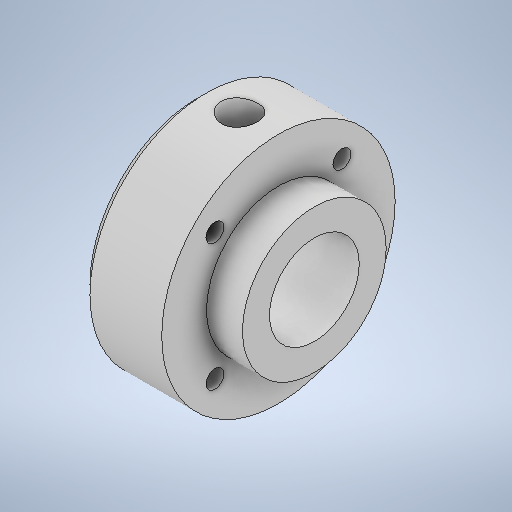
# Autodesk Inventor part: 08
Saved by Autodesk Inventor 2025.1 (Build 291241000, 241)
## iProperties
Created: 2024-09-17
Part Number: 08
Material: Generisch
Document SubType Name: Modeling
Designer: ffogue
Density: 1 g/cm^3
Appearance: Vorgabe
Author: ffogue
Autodesk Inventor part; units mm, degrees
ref_plane "YZ Plane" through (0, 0, 0) normal (1, 0, 0) x (0, 1, 0)
sketch "Sketch1" plane through (0, 0, 0) normal (0, 0, 1) x (1, 0, 0)
  line L0 (0, 0) -> (0, 13)
  line L1 (0, 13) -> (9, 13)
  line L2 (9, 13) -> (9, 8)
  line L3 (9, 8) -> (13, 8)
  line L4 (13, 8) -> (13, 0)
  line L5 (13, 0) -> (0, 0)
  dimension "d0" = 16
  dimension "d1" = 9
  dimension "d2" = 4
  dimension "d3" = 26
  constraints: 12 end point, 5 perpendicular, 1 vertical
  measures "d0" diameter of L3 L5
  measures "d1" distance of L0.end L1.end
  measures "d2" distance of L2.end L3.end
  measures "d3" diameter of L1 L5
revolve "Revolution1" add sketch "Sketch1" angle 360 about axis through (13, 0, 0) along (-1, 0, 0)
sketch "Sketch2" plane through (0, 0, 0) normal (-1, 0, 0) x (0, 0, 1)
  line L0 (0, 0) -> (7.0711, 7.0711) construction
  line L1 (0, 0) -> (13, 0) construction
  circle A0 centre (0, 0) radius 13 projected
  circle A1 centre (0, 0) radius 10 construction
  dimension "d6" = 20
  dimension "d5" = 45
  constraints: 4 end point, 2 horizontal alignment, 1 coincident, 1 horizontal, 4 other
  measures "d5" angle of L1 L0
hole "Hole1" at (0, 7.0711, 7.0711) direction (1, 0, 0) diameter 2 depth 9
pattern_circular "Circular Pattern1" count 4 over 360 about axis through (4.5, 0, 0) along (-1, 0, 0) of "Hole1"
sketch "Sketch3" plane through (0, 0, 0) normal (-1, 0, 0) x (0, 0, 1)
  circle A0 centre (0, 0) radius 13 projected
  point P0 (0, 0)
  constraints: 1 coincident
hole "Hole2" at (0, 0, 0) direction (1, 0, 0) diameter 10 depth 13
chamfer "Chamfer1" distance 1 angle 45 1 edges at (0, -13, 0)
ref_plane "Work Plane1" through (0, 0, 0) normal (0, 1, 0) x (-1, 0, 0)
sketch "Sketch4" plane through (0, 0, 0) normal (0, 1, 0) x (-1, 0, 0)
  line L0 (-13, -5) -> (-13, 5) projected
  line L1 (-13, -8) -> (-13, 8) projected
  line L2 (-7, 7) -> (-4.8162, 13)
  line L3 (-9, 13) -> (-1, 13) projected
  line L4 (-13, 5) -> (0, 5) projected
  point P0 (0, 0)
  dimension "d28" = 20
  dimension "d29" = 2
  dimension "d34" = 2
  constraints: 3 end point, 1 point on line
  measures "d28" angle of L1 L2
  measures "d29" horizontal distance of L3.start L2.start
  measures "d34" distance from line of L4 L2.start
ref_plane "Work Plane2" through (0, 0, 12.5) normal (0, 0, 1) x (1, 0, 0)
sketch "Sketch5" plane through (0, 0, 12.5) normal (0, 0, 1) x (1, 0, 0)
  circle A0 centre (4.8162, 0) radius 2
  point P0 (0, 0)
  dimension "d31" = 4
  constraints: 1 centre point, 1 coincident
  measures "d31" diameter of A0
sweep "Sweep1" cut profiles "Sketch5" path "Sketch4" path curves L2
body "Solid1"
